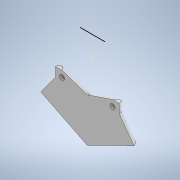
# Autodesk Inventor part: hank - name plate
Saved by Autodesk Inventor 2022 (Build 260153000, 153)
## iProperties
Created: 2021-01-16
Part Number: hank - name plate
Material: Generic
Document SubType Name: Modeling
Designer: chris
Density: 1 g/cm^3
Appearance: Default
Author: chris
Autodesk Inventor part; units mm, degrees
ref_plane "YZ Plane" through (0, 0, 0) normal (1, 0, 0) x (0, 1, 0)
ref_plane "XZ Plane" through (0, 0, 0) normal (0, 1, 0) x (-1, 0, 0)
ref_plane "XY Plane" through (0, 0, 0) normal (0, 0, 1) x (1, 0, 0)
sketch "Sketch1" plane through (0, 0, 0) normal (0, 0, 1) x (1, 0, 0)
  line L0 (-63.5, 63.5) -> (63.5, 63.5)
  line L1 (63.5, 63.5) -> (63.5, -63.5)
  line L2 (63.5, -63.5) -> (-63.5, -63.5)
  line L3 (-63.5, -63.5) -> (-63.5, 63.5)
  circle A0 centre (-57.15, 57.15) radius 1.524
  circle A1 centre (57.15, 57.15) radius 1.524
  line L4 (63.5, 0) -> (-63.5, 0)
  circle A2 centre (-57.15, -57.15) radius 1.524
  circle A3 centre (57.15, -57.15) radius 1.524
  point P0 (0, 0)
  point P1 (0, 63.5)
  dimension "d0" = 127
  dimension "d1" = 127
  dimension "d2" = 127
  dimension "d3" = 3.048
  dimension "d4" = 3.048
  dimension "d5" = 6.35
  dimension "d6" = 6.35
  dimension "d7" = 6.35
  dimension "d8" = 6.35
  constraints: 10 end point, 4 centre point, 3 midpoint, 2 perpendicular, 2 symmetric about line, 1 horizontal, 1 horizontal alignment, 1 vertical alignment, 2 other
  measures "d0" distance of L0.start L0.end
  measures "d1" distance of L0.end L1.end
  measures "d2" distance of L1.end L2.end
  measures "d3" diameter of A0
  measures "d4" diameter of A1
  measures "d5" distance from line of L3 A0.centre
  measures "d6" distance from line of L0 A0.centre
  measures "d7" distance from line of L0 A1.centre
  measures "d8" distance from line of L1 A1.centre
extrude "Extrusion1" add sketch "Sketch1" along normal blind 3.175
sketch "Sketch2" plane through (0, 0, 3.175) normal (0, 0, 1) x (1, 0, 0)
  circle A0 centre (0, 0) radius 3.81
  circle A1 centre (-15.494, 15.494) radius 1.524
  circle A2 centre (15.494, 15.494) radius 1.524
  circle A3 centre (-15.494, -15.494) radius 1.524
  circle A4 centre (15.494, -15.494) radius 1.524
  line L0 (-15.494, 15.494) -> (15.494, 15.494)
  line L1 (-15.494, -15.494) -> (-15.494, 15.494)
  point P0 (0, 15.494)
  point P1 (-15.494, 0)
  dimension "d11" = 7.62
  dimension "d12" = 3.048
  dimension "d13" = 3.048
  dimension "d14" = 3.048
  dimension "d15" = 3.048
  dimension "d16" = 30.988
  dimension "d21" = 30.988
  dimension "d22" = 30.988
  constraints: 5 centre point, 4 end point, 3 vertical alignment, 2 midpoint, 1 coincident, 1 horizontal, 1 horizontal alignment, 1 vertical
  measures "d11" diameter of A0
  measures "d12" diameter of A1
  measures "d13" diameter of A2
  measures "d14" diameter of A3
  measures "d15" diameter of A4
  measures "d16" distance of L0.end L0.start
  measures "d21" distance of L1.start L0.start
  measures "d22" distance of A4.centre L0.end
extrude "Extrusion2" cut sketch "Sketch2" against normal blind 25.4
fillet "Fillet1" radius 3.175 4 edges at (0, 63.5, 0) (-63.5, 0, 0) (0, -63.5, 0) (63.5, 0, 0)
sketch "Sketch4" plane through (0, 0, 0) normal (0, 0, -1) x (-1, 0, 0)
  circle A0 centre (0, 0) radius 3.81
  line L0 (0, 0) -> (50.8, 0)
  line L1 (60.325, 60.325) -> (60.325, -60.325)
  line L2 (-60.325, 60.325) -> (60.325, 60.325)
  line L3 (0, 60.325) -> (60.325, 60.325)
  line L4 (63.5, 63.5) -> (63.5, -63.5)
  line L5 (60.325, 60.325) -> (60.325, 47.625)
  line L6 (25.4, 0) -> (25.4, 47.625)
  circle A1 centre (25.4, 47.625) radius 3.75
  circle A2 centre (50.8, 0) radius 3.75
  circle A3 centre (25.4, -47.625) radius 3.75
  line L7 (25.4, 47.625) -> (50.8, 0)
  line L8 (50.8, 0) -> (25.4, -47.625)
  line L9 (27.054412, 48.507353) -> (52.925, 0)
  line L10 (52.925, 0) -> (27.054412, -48.507353)
  line L11 (23.745588, 46.742647) -> (48.675, 0)
  line L12 (48.675, 0) -> (23.745588, -46.742647)
  circle A4 centre (15.494, 15.494) radius 1.524
  line L13 (15.494, 0) -> (7.747, -13.418198)
  line L14 (7.747, -13.418198) -> (-7.747, -13.418198)
  line L15 (-7.747, -13.418198) -> (-15.494, 0)
  line L16 (-15.494, 0) -> (-7.747, 13.418198)
  line L17 (-7.747, 13.418198) -> (7.747, 13.418198)
  line L18 (7.747, 13.418198) -> (15.494, 0)
  line L19 (0, 60.325) -> (0, 13.418198)
  line L20 (0, 0) -> (-50.8, 0)
  line L21 (-25.4, 0) -> (-25.4, 47.625)
  circle A5 centre (-25.4, 47.625) radius 3.75
  circle A6 centre (-50.8, 0) radius 3.75
  circle A7 centre (-25.4, -47.625) radius 3.75
  line L22 (-25.4, 47.625) -> (-50.8, 0)
  line L23 (-50.8, 0) -> (-25.4, -47.625)
  line L24 (-27.054412, 48.507353) -> (-52.925, 0)
  line L25 (-52.925, 0) -> (-27.054412, -48.507353)
  line L26 (-23.745588, 46.742647) -> (-48.675, 0)
  line L27 (-48.675, 0) -> (-23.745588, -46.742647)
  circle A8 centre (-15.494, 15.494) radius 1.524
  point P0 (-25.4, 43.875)
  point P1 (-28.582692, 45.641828)
  point P2 (-50.926132, 3.747878)
  point P3 (-50.926132, -3.747878)
  point P4 (-28.582692, -45.641828)
  point P5 (-25.273868, -43.877122)
  point P6 (-47.617308, -1.983172)
  point P7 (-47.617308, 1.983172)
  point P8 (-25.4, 43.640625)
  point P9 (50.926132, 3.747878)
  point P10 (28.582692, 45.641828)
  point P11 (25.4, 43.875)
  point P12 (25.4, 43.640625)
  point P13 (47.617308, 1.983172)
  point P14 (47.617308, -1.983172)
  point P15 (25.273868, -43.877122)
  point P16 (28.582692, -45.641828)
  point P17 (50.926132, -3.747878)
  dimension "d24" = 50.8
  dimension "d25" = 12.7
  dimension "d26" = 7.5
  dimension "d27" = 7.5
  dimension "d28" = 1.875
  dimension "d29" = 1.875
  constraints: 50 end point, 14 symmetric about line, 7 centre point, 5 coincident, 3 midpoint, 2 perpendicular, 2 point on line, 1 horizontal alignment, 1 vertical, 20 other
  measures "d24" distance of L0.start L0.end
  measures "d25" distance of L1.start L5.end
  measures "d26" diameter of A1
  measures "d27" diameter of A2
  measures "d28" distance between parallel lines of L7 L9
  measures "d29" distance between parallel lines of L7 L11
extrude "Extrusion3" cut sketch "Sketch4" against normal blind 1 contours L0 L13 L14 L15 L20 A0 | A0 L20 L16 L17 L18 L0 | L11 A2 L7 L0 | L12 A2 L0 | L0 A2 L11 | L0 L8 A2 L12 | L7 A2 L9 L10 L8 | L11 L6 A1 L7 A2 | A2 L8 A3 L12 | L7 A1 L9 A2 | A2 L10 A3 L8 | A3 | A2 L10 L9 | L7 L6 A1 | A1 L6 L7 | A6 L27 L20 | L20 L26 A6 | L26 A6 L22 A5 L21 | L27 A6 L23 L20 | L20 L22 A6 L26 | L27 A7 L23 A6 | A5 L22 L21 | L21 L22 A5 | L23 A6 L25 L24 L22 | A6 L24 A5 L22 | L23 A7 L25 A6 | A7 | L24 L25 A6
sketch "Sketch5" plane through (0, 0, 0) normal (0, 0, -1) x (-1, 0, 0)
  line L0 (-7.747, 13.418198) -> (7.747, 13.418198)
  line L1 (7.747, 13.418198) -> (-7.747, 13.418198)
  point P0 (0, 0)
  constraints: 2 end point, 1 horizontal
sketch "Sketch6" plane through (0, 0, 0) normal (0, 0, -1) x (-1, 0, 0)
  line L0 (15.494, 0) -> (7.747, -13.418198)
  line L1 (7.747, -13.418198) -> (-7.747, -13.418198)
  line L2 (-7.747, -13.418198) -> (-15.494, 0)
  line L3 (-15.494, 0) -> (-7.747, 13.418198)
  line L4 (-7.747, 13.418198) -> (7.747, 13.418198)
  line L5 (7.747, 13.418198) -> (15.494, 0)
  arc A0 (-50.926132, 3.747878) -> (-50.926132, -3.747878) centre (-50.8, 0) ccw
  line L6 (-50.926132, 3.747878) -> (-28.582692, 45.641828)
  arc A1 (-25.4, 43.875) -> (-28.582692, 45.641828) centre (-25.4, 47.625) ccw
  line L7 (-25.4, 43.875) -> (-25.4, 43.640625)
  line L8 (-25.4, 43.640625) -> (-47.617308, 1.983172)
  arc A2 (-47.617308, -1.983172) -> (-47.617308, 1.983172) centre (-50.8, 0) ccw
  line L9 (-47.617308, -1.983172) -> (-25.273868, -43.877122)
  arc A3 (-28.582692, -45.641828) -> (-25.273868, -43.877122) centre (-25.4, -47.625) ccw
  line L10 (-28.582692, -45.641828) -> (-50.926132, -3.747878)
  line L11 (25.4, 43.640625) -> (25.4, 43.875)
  arc A4 (28.582692, 45.641828) -> (25.4, 43.875) centre (25.4, 47.625) ccw
  line L12 (28.582692, 45.641828) -> (50.926132, 3.747878)
  arc A5 (50.926132, -3.747878) -> (50.926132, 3.747878) centre (50.8, 0) ccw
  line L13 (50.926132, -3.747878) -> (28.582692, -45.641828)
  arc A6 (25.273868, -43.877122) -> (28.582692, -45.641828) centre (25.4, -47.625) ccw
  line L14 (25.273868, -43.877122) -> (47.617308, -1.983172)
  arc A7 (47.617308, 1.983172) -> (47.617308, -1.983172) centre (50.8, 0) ccw
  line L15 (47.617308, 1.983172) -> (25.4, 43.640625)
  circle A8 centre (-57.15, 57.15) radius 1.524
  circle A9 centre (57.15, 57.15) radius 1.524
  circle A10 centre (-57.15, -57.15) radius 1.524
  circle A11 centre (57.15, -57.15) radius 1.524
  circle A12 centre (-15.494, -15.494) radius 1.524
  circle A13 centre (-15.494, 15.494) radius 1.524
  circle A14 centre (15.494, -15.494) radius 1.524
  circle A15 centre (15.494, 15.494) radius 1.524
  line L16 (-60.325, -60.325) -> (-60.325, 60.325)
  line L17 (60.325, -60.325) -> (-60.325, -60.325)
  line L18 (60.325, 60.325) -> (60.325, -60.325)
  line L19 (-60.325, 60.325) -> (60.325, 60.325)
  line L20 (-15.494, -11.755967) -> (0, -17.018)
  line L21 (0, -17.018) -> (15.494, -11.755967)
  line L22 (15.494, -11.755967) -> (23.635294, -22.930147)
  line L23 (-23.635294, -22.930147) -> (-15.494, -11.755967)
  line L24 (-15.494, -11.755967) -> (-19.564647, -11.755967)
  line L25 (-19.564647, -11.755967) -> (-19.564647, -17.343057)
  line L26 (7.747, -13.418198) -> (15.494, 0)
  line L27 (15.494, -11.755967) -> (19.564647, -11.755967)
  line L28 (19.564647, -11.755967) -> (19.564647, -17.343057)
  line L29 (-21.75005, -21.772113) -> (-5.022552, -21.772113) construction
  line L30 (-5.022552, -21.772113) -> (-5.022552, -26.820056) construction
  line L31 (-5.022552, -26.820056) -> (-21.75005, -26.820056) construction
  line L32 (-21.75005, -26.820056) -> (-21.75005, -21.772113) construction
  line L33 (-63.5, 63.5) -> (63.5, 63.5)
  line L34 (-63.5, -63.5) -> (-63.5, 63.5)
  line L35 (63.5, 63.5) -> (63.5, -63.5)
  line L36 (63.5, -63.5) -> (-63.5, -63.5)
  line L37 (-15.494, -11.755967) -> (-28.582692, -29.720605)
  line L38 (-28.582692, -29.720605) -> (0, -43.877122)
  line L39 (15.494, -11.755967) -> (28.582692, -29.720605)
  line L40 (28.582692, -29.720605) -> (0, -43.877122)
  line L41 (-13.929875, -30.027113) -> (-16.00366, -30.027113)
  line L42 (-16.00366, -30.027113) -> (-16.00366, -26.367887)
  line L43 (-16.00366, -26.367887) -> (-18.819993, -26.367887)
  line L44 (-18.819993, -26.367887) -> (-18.819993, -30.027113)
  line L45 (-18.819993, -30.027113) -> (-20.893777, -30.027113)
  line L46 (-20.893777, -30.027113) -> (-20.893777, -21.772113)
  line L47 (-20.893777, -21.772113) -> (-18.819993, -21.772113)
  line L48 (-18.819993, -21.772113) -> (-18.819993, -24.795825)
  line L49 (-18.819993, -24.795825) -> (-16.00366, -24.795825)
  line L50 (-16.00366, -24.795825) -> (-16.00366, -21.772113)
  line L51 (-16.00366, -21.772113) -> (-13.929875, -21.772113)
  line L52 (-13.929875, -21.772113) -> (-13.929875, -30.027113)
  line L53 (-10.324166, -30.027113) -> (-12.284227, -30.027113)
  line L54 (-12.284227, -30.027113) -> (-12.284227, -27.846295)
  line L55 (-12.284227, -27.846295) -> (-10.324166, -27.846295)
  line L56 (-10.324166, -27.846295) -> (-10.324166, -30.027113)
  line L57 (-9.561549, -30.027113) -> (-6.771974, -21.772113)
  line L58 (-6.771974, -21.772113) -> (-4.51088, -21.772113)
  line L59 (-4.51088, -21.772113) -> (-1.721305, -30.027113)
  line L60 (-1.721305, -30.027113) -> (-3.855297, -30.027113)
  line L61 (-3.855297, -30.027113) -> (-4.370398, -28.341327)
  line L62 (-4.370398, -28.341327) -> (-6.965973, -28.341327)
  line L63 (-6.965973, -28.341327) -> (-7.487764, -30.027113)
  line L64 (-7.487764, -30.027113) -> (-9.561549, -30.027113)
  line L65 (-4.825293, -26.842851) -> (-5.668186, -24.113483)
  line L66 (-5.668186, -24.113483) -> (-6.517768, -26.842851)
  line L67 (-6.517768, -26.842851) -> (-4.825293, -26.842851)
  line L68 (0.994683, -30.027113) -> (-0.965378, -30.027113)
  line L69 (-0.965378, -30.027113) -> (-0.965378, -27.846295)
  line L70 (-0.965378, -27.846295) -> (0.994683, -27.846295)
  line L71 (0.994683, -27.846295) -> (0.994683, -30.027113)
  line L72 (9.717957, -30.027113) -> (7.724448, -30.027113)
  line L73 (7.724448, -30.027113) -> (4.540186, -24.274034)
  line L74 (4.540186, -24.274034) -> (4.540186, -30.027113)
  line L75 (4.540186, -30.027113) -> (2.647021, -30.027113)
  line L76 (2.647021, -30.027113) -> (2.647021, -21.772113)
  line L77 (2.647021, -21.772113) -> (5.18908, -21.772113)
  line L78 (5.18908, -21.772113) -> (7.824793, -26.50168)
  line L79 (7.824793, -26.50168) -> (7.824793, -21.772113)
  line L80 (7.824793, -21.772113) -> (9.717957, -21.772113)
  line L81 (9.717957, -21.772113) -> (9.717957, -30.027113)
  line L82 (13.290218, -30.027113) -> (11.330157, -30.027113)
  line L83 (11.330157, -30.027113) -> (11.330157, -27.846295)
  line L84 (11.330157, -27.846295) -> (13.290218, -27.846295)
  line L85 (13.290218, -27.846295) -> (13.290218, -30.027113)
  line L86 (22.174043, -30.027113) -> (19.665433, -30.027113)
  line L87 (19.665433, -30.027113) -> (17.424408, -26.67561)
  line L88 (17.424408, -26.67561) -> (17.016341, -27.237539)
  line L89 (17.016341, -27.237539) -> (17.016341, -30.027113)
  line L90 (17.016341, -30.027113) -> (14.942556, -30.027113)
  line L91 (14.942556, -30.027113) -> (14.942556, -21.772113)
  line L92 (14.942556, -21.772113) -> (17.016341, -21.772113)
  line L93 (17.016341, -21.772113) -> (17.016341, -25.458098)
  line L94 (17.016341, -25.458098) -> (19.665433, -21.772113)
  line L95 (19.665433, -21.772113) -> (22.05363, -21.772113)
  line L96 (22.05363, -21.772113) -> (19.110194, -25.60527)
  line L97 (19.110194, -25.60527) -> (22.174043, -30.027113)
  point P0 (0, 0)
  point P1 (15.494, -11.755967)
  constraints: 26 end point, 1 horizontal, 1 midpoint, 2 other
extrude "Extrusion4" cut sketch "Sketch6" against normal through all contours L0 L1 L2 L3 L4 L5 | L6 A1 L7 L8 A2 L9 A3 L10 A0 | L11 A4 L12 A5 L13 A6 L14 A7 L15 | A8 | A9 | A10 | A11 | A12 | A13 | A14 | A15 | L16 L19 L18 L17 | L33 L35 L36 L34
extrude "Extrusion6" cut sketch "Sketch6" against normal blind 1 contours L41 L42 L43 L44 L45 L46 L47 L48 L49 L50 L51 L52 | L53 L54 L55 L56 | L57 L58 L59 L60 L61 L62 L63 L64 | L68 L69 L70 L71 | L72 L73 L74 L75 L76 L77 L78 L79 L80 L81 | L82 L83 L84 L85 | L86 L87 L88 L89 L90 L91 L92 L93 L94 L95 L96 L97
fillet "Fillet2" radius 3.175 8 edges at (19.5646, -14.5495, 0) (-19.5646, -14.5495, 0) (7.747, -14.387, 0) (-7.747, -14.387, 0) (-24.0737, -23.5318, 0) (24.0737, -23.5318, 0) (14.2913, -36.7989, 0) (-14.2913, -36.7989, 0)
body "Solid1"
